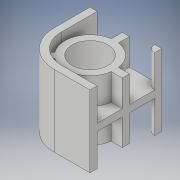
# Autodesk Inventor part: Bent beam base-90
Saved by Autodesk Inventor 2019.3 (Build 233278000, 278)
## iProperties
Created: 2019-01-29
Part Number: Bent beam base-90
Material: Generic
Document SubType Name: Modeling
Designer: Varga Daniel
Density: 1 g/cm^3
Appearance: Default
Hole_height: 8,400 mm
Beam_angle: 90,00 deg
First_hole_pos: 5,000 mm
Author: Varga Daniel
Autodesk Inventor part; units mm, degrees
ref_plane "YZ Plane" through (0, 0, 0) normal (1, 0, 0) x (0, 1, 0)
ref_plane "XZ Plane" through (0, 0, 0) normal (0, 1, 0) x (-1, 0, 0)
ref_plane "XY Plane" through (0, 0, 0) normal (0, 0, 1) x (1, 0, 0)
derived "Base_part.ipt"
sketch "Beam_sketch" plane through (0, 0, 0) normal (0, 1, 0) x (-1, 0, 0)
  line L0 (5, 0) -> (25, 0)
  line L1 (30, 5) -> (30, 25)
  line L2 (25, 30) -> (5, 30)
  line L3 (0, 25) -> (0, 5)
  line L4 (5, 29) -> (25, 29)
  line L5 (29, 25) -> (29, 5)
  line L6 (25, 1) -> (5, 1)
  line L7 (1, 5) -> (1, 25)
  circle A0 centre (5, 5) radius 2.5
  circle A1 centre (5, 5) radius 3.5
  arc A2 (25, 0) -> (30, 5) centre (25, 5) ccw
  arc A3 (30, 25) -> (25, 30) centre (25, 25) ccw
  arc A4 (5, 30) -> (0, 25) centre (5, 25) ccw
  arc A5 (0, 5) -> (5, 0) centre (5, 5) ccw
  arc A6 (1, 5) -> (5, 1) centre (5, 5) ccw
  arc A7 (5, 29) -> (1, 25) centre (5, 25) ccw
  arc A8 (29, 25) -> (25, 29) centre (25, 25) ccw
  arc A9 (25, 1) -> (29, 5) centre (25, 5) ccw
  line L8 (49.1041, 15) -> (-27.081, 15) construction
  line L9 (31.1478, 10) -> (-2.4877, 10) construction
  line L10 (-2.8604, 5) -> (35.495, 5) construction
  line L11 (5, -2.5736) -> (5, 36.7522) construction
  line L12 (15, -1.4978) -> (15, 34.8784) construction
  line L13 (1.5359, 5.5) -> (1, 5.5)
  line L14 (1.5359, 4.5) -> (1.0314, 4.5)
  line L15 (28.9686, 4.5) -> (8.4641, 4.5)
  line L16 (29, 5.5) -> (8.4641, 5.5)
  line L17 (4.5, 1.5359) -> (4.5, 1.0314)
  line L18 (5.5, 1.5359) -> (5.5, 1)
  line L19 (29, 10.5) -> (1, 10.5)
  line L20 (29, 9.5) -> (1, 9.5)
  line L21 (4.5, 28.9686) -> (4.5, 10.5)
  line L22 (4.5, 9.5) -> (4.5, 8.4641)
  line L23 (5.5, 29) -> (5.5, 10.5)
  line L24 (5.5, 9.5) -> (5.5, 8.4641)
  point P0 (0, 0)
  point P1 (30, 30)
  point P2 (0, 30)
derived "Connector_pin_base.ipt"
sketch "Pin_base_sketch" plane through (0, 0, 0) normal (0, 0, 1) x (1, 0, 0)
  line L0 (0, 0) -> (23.0918, 0) construction
  line L1 (0, 0) -> (0, 6.22) construction
  line L2 (0, 3.75) -> (0.563, 3.75)
  line L3 (0.863, 3.45) -> (0.863, 2.475)
  line L4 (0.863, 2.475) -> (9.988, 2.475)
  line L5 (9.988, 2.475) -> (9.988, 0)
  line L6 (0, 0) -> (0, 3.75)
  line L7 (0, 0) -> (9.988, 0)
  line L8 (9.288, 2.475) -> (9.288, 2.6)
  line L9 (9.988, 2.475) -> (9.988, 2.4774)
  arc A0 (9.988, 2.4774) -> (9.8454, 2.7031) centre (9.738, 2.4774) ccw
  arc A1 (9.8454, 2.7031) -> (9.288, 2.6) centre (9.6379, 2.267) ccw
  line L10 (9.8454, 2.7031) -> (9.8454, -0.0362) construction
  line L11 (8.9584, 2.75) -> (10.3858, 2.75) construction
  arc A2 (0.863, 3.45) -> (0.563, 3.75) centre (0.563, 3.45) ccw
  line L12 (0.863, 2.475) -> (0.863, 0)
  line L13 (-0.863, 2.475) -> (-0.863, 0)
  line L14 (-0.863, 3.45) -> (-0.863, 2.475)
  arc A3 (-0.563, 3.75) -> (-0.863, 3.45) centre (-0.563, 3.45) ccw
  line L15 (0, 3.75) -> (-0.563, 3.75)
  line L16 (0, 0) -> (-23.0918, 0) construction
  line L17 (0, 0) -> (-9.988, 0)
  line L18 (-0.863, 2.475) -> (-9.988, 2.475)
  line L19 (-9.288, 2.475) -> (-9.288, 2.6)
  arc A4 (-9.288, 2.6) -> (-9.8454, 2.7031) centre (-9.6379, 2.267) ccw
  arc A5 (-9.8454, 2.7031) -> (-9.988, 2.4774) centre (-9.738, 2.4774) ccw
  line L20 (-9.988, 2.475) -> (-9.988, 2.4774)
  line L21 (-8.9584, 2.75) -> (-10.3858, 2.75) construction
  line L22 (-9.8454, 2.7031) -> (-9.8454, -0.0362) construction
  line L23 (-9.988, 2.475) -> (-9.988, 0)
  line L24 (9.638, 3.1946) -> (9.638, -1.2485) construction
sketch "Sketch2" plane through (0, 0, 0) normal (0, 1, 0) x (-1, 0, 0)
  line L0 (-9.8186, -6.0609) -> (-9.8186, -6.0609)
  line L1 (0.1814, -1.0609) -> (0.1814, -6.0609)
  line L2 (-0.8186, -1.0609) -> (-0.8186, -6.0609)
  line L3 (-8.8186, -6.0609) -> (-8.8186, -6.0609)
  line L4 (-4.8186, -1.0609) -> (-4.8186, -21.0609) construction
  line L5 (-9.8186, -6.0609) -> (-9.8186, -6.0609)
  line L6 (-9.8186, -5.0609) -> (-9.8186, -5.0609)
  line L7 (-4.8186, -1.0609) -> (5.7458, -1.0609) construction
  line L8 (-9.8186, -6.0609) -> (18.8493, 22.6071) construction
  arc A0 (-8.8186, -6.0609) -> (-9.8186, -5.0609) centre (-9.8186, -6.0609) ccw
  arc A1 (0.1814, -1.0609) -> (-4.8186, 3.9391) centre (-4.8186, -1.0609) ccw
  line L9 (-4.8186, 3.9391) -> (-9.8186, 3.9391)
  line L10 (-4.8186, 2.9391) -> (-9.8186, 2.9391)
  arc A2 (-0.8186, -1.0609) -> (-1.6589, 1.3918) centre (-4.8186, -1.0609) ccw
  circle A3 centre (-4.8186, -1.0609) radius 2.5
  arc A4 (-2.0156, 1.0351) -> (-2.7227, 1.7422) centre (-4.8186, -1.0609) ccw
  line L11 (-4.3186, -4.525) -> (-4.3186, -6.0609)
  line L12 (-5.3186, -6.0609) -> (-5.3186, -4.525)
  line L13 (-8.2827, -1.5609) -> (-9.8186, -1.5609)
  line L14 (-9.8186, -0.5609) -> (-8.2827, -0.5609)
  line L15 (-1.6589, 1.3918) -> (-2.0156, 1.0351)
  line L16 (-2.366, 2.0989) -> (-2.7227, 1.7422)
  circle A5 centre (5, 5) radius 2.5 construction
  circle A6 centre (5, 5) radius 3.5 construction
  line L17 (-9.8186, -6.0609) -> (0.1814, -6.0609)
  line L18 (-9.8186, 3.9391) -> (-9.8186, -6.0609)
  arc A7 (-4.3186, -4.525) -> (-2.0156, 1.0351) centre (-4.8186, -1.0609) ccw
  arc A8 (-2.7227, 1.7422) -> (-4.3186, -4.525) centre (-4.8186, -1.0609) ccw
  arc A9 (-1.6589, 1.3918) -> (-2.366, 2.0989) centre (-4.8186, -1.0609) ccw
  arc A10 (-2.366, 2.0989) -> (-4.8186, 2.9391) centre (-4.8186, -1.0609) ccw
  dimension "d7" = 1
  dimension "d9" = 90
  dimension "d10" = 1
  dimension "d11" = 1
  dimension "d14" = 1
  dimension "d16" = 5
  dimension "d17" = 4
  dimension "d18" = 5
  dimension "d19" = 7
  dimension "d83" = 1
  dimension "d84" = 1
  dimension "d96" = 1
  dimension "d105" = 5
  dimension "d106" = 7
  dimension "d107" = 1
  dimension "d108" = 10
  dimension "d109" = 5
  dimension "d110" = 5
  constraints: 38 end point, 23 point on circle, 13 parallel, 9 centre point, 9 point on line, 6 tangent, 4 coincident, 3 vertical, 2 perpendicular, 6 other
  measures "d7" distance between parallel lines of L1 L2
  measures "d9" angle of L4 L7
  measures "d10" distance between parallel lines of L5 L6
  measures "d11" radius of A0
  measures "d14" distance between parallel lines of L10 L9
  measures "d16" radius of A1
  measures "d17" radius of A2
  measures "d18" diameter of A3
  measures "d19" diameter of A4
  measures "d83" distance between parallel lines of L12 L11
  measures "d84" distance between parallel lines of L14 L13
  measures "d96" distance between parallel lines of L16 L15
  measures "d105" diameter of A5
  measures "d106" diameter of A6
  measures "d107" distance between parallel lines of L3 L0
  measures "d108" distance between parallel lines of L1 L0
  measures "d109" distance from line of L4.start L17
  measures "d110" distance from line of A1.centre L18
ref_plane "Work Plane1" through (9.8186, 0, -6.0609) normal (0, -1, 0) x (-1, 0, 0)
extrude "Extrusion13" add sketch "Sketch2" along normal mid plane 8.4 contours L17 L12 A8 L11 | L15 A4 L16 A9 | A8 A4 A7 | L14 A8 L13 L18
extrude "Extrusion14" add sketch "Sketch2" along normal mid plane 10 contours L1 L17 L2 A2 A9 A10 L10 L18 L9 A1 | L17 L18 A0
extrude "Extrusion15" add sketch "Sketch2" along normal mid plane 1 contours L17 L11 A7 L15 A2 L2 | L10 A10 L16 A8 L14 L18 | L17 A0 L18 L13 A8 L12
ref_plane "Work Plane2" through (4.8186, -4.2, -0.5609) normal (1, 0, 0) x (0, 0, -1)
ref_plane "Work Plane3" through (5.3186, 4.2, -1.0609) normal (0, 0, -1) x (-1, 0, 0)
sketch "Sketch5" plane through (-0.1814, -5, -1.0609) normal (-1, 0, 0) x (0, 0, 1)
  arc A0 (0, 8.75) -> (0, 1.25) centre (0, 5) ccw
  line L0 (0, -2.244) -> (0, 13.4639) projected
  arc A1 (0, 1.25) -> (0, 8.75) centre (0, 5) ccw
  point P0 (1.0609, 5)
  dimension "d133" = 7.5
  constraints: 4 point on circle, 2 centre point, 2 point on line, 1 coincident
  measures "d133" diameter of A0
extrude "Extrusion16" [suppressed]
extrude "Extrusion17" [suppressed]
sketch "Sketch6" plane through (4.8186, 5, 3.9391) normal (0, 0, 1) x (1, 0, 0)
  line L0 (0, 3.4639) -> (0, -12.244) projected
  arc A0 (0, -8.75) -> (0, -1.25) centre (0, -5) ccw
  arc A1 (0, -1.25) -> (0, -8.75) centre (0, -5) ccw
  point P0 (-4.8186, -5)
  dimension "d142" = 7.5
  constraints: 4 point on circle, 2 centre point, 2 point on line, 1 coincident
  measures "d142" diameter of A0
extrude "Extrusion18" [suppressed]
extrude "Extrusion19" [suppressed]
sketch "Sketch4" plane through (0, 0, 0) normal (0, 0, 1) x (1, 0, 0)
  arc A0 (0.863, 3.45) -> (0.563, 3.75) centre (0.563, 3.45) ccw construction
  line L0 (0.863, 3.45) -> (0.863, 2.475) construction
  line L1 (0.863, 2.475) -> (0.863, 0) construction
  line L2 (0, 0) -> (9.988, 0) construction
  line L3 (0, 0) -> (0, 6.22) construction
  line L4 (0, 0) -> (0, 3.75) construction
  line L5 (0, 3.75) -> (0.563, 3.75) construction
  dimension "d130" = 0.863
  dimension "d131" = 3.75
  dimension "d132" = 0.3
  measures "d130" distance between parallel lines of L1 L3
  measures "d131" distance between parallel lines of L2 L5
  measures "d132" radius of A0
equation "\"d10\" = d7"
equation "\"d11\" = d7"
equation "\"d14\" = d7"
equation "\"d17\" = d16 - d7"
equation "\"d83\" = Inner_route_thickness"
equation "\"d84\" = Inner_route_thickness"
equation "\"Beam_angle\" = 90deg"
equation "\"First_hole_pos\" = 5"
equation "\"Inner_route_thickness\" = 1"
body "Solid3"
